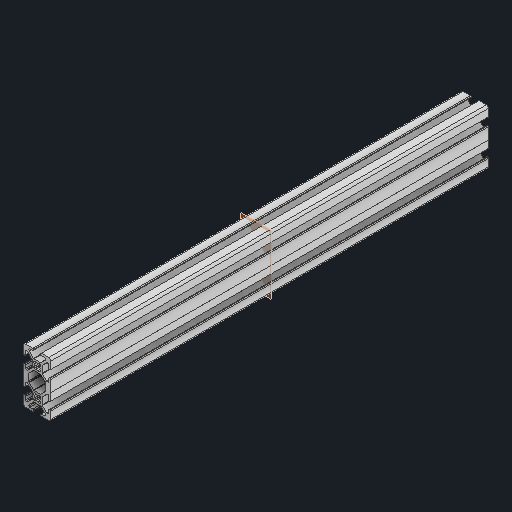
# Autodesk Inventor part: 20-2020-285
Saved by Autodesk Inventor 2026.2 (Build 302298000, 298)
## iProperties
Created: 2024-06-13
Part Number: 20-2020-285
Material: Generic
Document SubType Name: Modeling
Designer: mumin
Density: 1 g/cm^3
Appearance: Default
Author: mumin
Autodesk Inventor part; units mm, degrees
ref_plane "YZ Plane" through (0, 0, 0) normal (1, 0, 0) x (0, 1, 0)
ref_plane "XZ Plane" through (0, 0, 0) normal (0, 1, 0) x (-1, 0, 0)
sketch "Sketch1" plane through (0, 0, 0) normal (0, 0, 1) x (1, 0, 0)
  arc A0 (-10, -8.5) -> (-8.5, -10) centre (-8.5, -8.5) ccw
  line L0 (-8.5, -10) -> (-3.138, -10)
  arc A1 (-3.138, -10) -> (-2.63, -9.492) centre (-3.138, -9.492) ccw
  line L1 (-2.63, -9.492) -> (-2.63, -9.008)
  arc A2 (-2.63, -9.008) -> (-3.138, -8.5) centre (-3.138, -9.008) ccw
  line L2 (-3.138, -8.5) -> (-5.487, -8.5)
  arc A3 (-5.995, -7.992) -> (-5.487, -8.5) centre (-5.487, -7.992) ccw
  line L3 (-5.995, -7.992) -> (-5.995, -7.2662)
  arc A4 (-5.8462, -6.907) -> (-5.995, -7.2662) centre (-5.487, -7.2662) ccw
  line L4 (-5.8462, -6.907) -> (-2.743, -3.8038)
  arc A5 (-2.3838, -3.655) -> (-2.743, -3.8038) centre (-2.3838, -4.163) ccw
  line L5 (-2.3838, -3.655) -> (2.3841, -3.655)
  arc A6 (2.7433, -3.8038) -> (2.3841, -3.655) centre (2.3841, -4.163) ccw
  line L6 (2.7433, -3.8038) -> (5.8462, -6.9067)
  arc A7 (5.995, -7.2659) -> (5.8462, -6.9067) centre (5.487, -7.2659) ccw
  line L7 (5.995, -7.2659) -> (5.995, -7.992)
  arc A8 (5.487, -8.5) -> (5.995, -7.992) centre (5.487, -7.992) ccw
  line L8 (5.487, -8.5) -> (3.138, -8.5)
  arc A9 (3.138, -8.5) -> (2.63, -9.008) centre (3.138, -9.008) ccw
  line L9 (2.63, -9.008) -> (2.63, -9.492)
  arc A10 (2.63, -9.492) -> (3.138, -10) centre (3.138, -9.492) ccw
  line L10 (3.138, -10) -> (8.5, -10)
  arc A11 (8.5, -10) -> (10, -8.5) centre (8.5, -8.5) ccw
  line L11 (10, -8.5) -> (10, -3.138)
  arc A12 (10, -3.138) -> (9.492, -2.63) centre (9.492, -3.138) ccw
  line L12 (9.492, -2.63) -> (9.008, -2.63)
  arc A13 (9.008, -2.63) -> (8.5, -3.138) centre (9.008, -3.138) ccw
  line L13 (8.5, -3.138) -> (8.5, -5.487)
  arc A14 (7.992, -5.995) -> (8.5, -5.487) centre (7.992, -5.487) ccw
  line L14 (7.992, -5.995) -> (7.2662, -5.995)
  arc A15 (6.907, -5.8462) -> (7.2662, -5.995) centre (7.2662, -5.487) ccw
  line L15 (6.907, -5.8462) -> (3.8038, -2.743)
  arc A16 (3.655, -2.3838) -> (3.8038, -2.743) centre (4.163, -2.3838) ccw
  line L16 (3.655, -2.3838) -> (3.655, 2.3841)
  arc A17 (3.8038, 2.7433) -> (3.655, 2.3841) centre (4.163, 2.3841) ccw
  line L17 (3.8038, 2.7433) -> (6.9067, 5.8462)
  arc A18 (7.2659, 5.995) -> (6.9067, 5.8462) centre (7.2659, 5.487) ccw
  line L18 (7.2659, 5.995) -> (7.992, 5.995)
  arc A19 (8.5, 5.487) -> (7.992, 5.995) centre (7.992, 5.487) ccw
  line L19 (8.5, 5.487) -> (8.5, 3.138)
  arc A20 (8.5, 3.138) -> (9.008, 2.63) centre (9.008, 3.138) ccw
  line L20 (9.008, 2.63) -> (9.492, 2.63)
  arc A21 (9.492, 2.63) -> (10.0003, 3.1379) centre (9.4923, 3.138) ccw
  line L21 (10.0003, 3.1379) -> (10.0003, 8.4999)
  line L22 (5.995, 12.0036) -> (5.995, 7.2663)
  arc A22 (5.8462, 6.9071) -> (5.995, 7.2663) centre (5.487, 7.2663) ccw
  line L23 (5.8462, 6.9071) -> (2.7429, 3.8038)
  arc A23 (2.3837, 3.655) -> (2.7429, 3.8038) centre (2.3837, 4.163) ccw
  line L24 (2.3837, 3.655) -> (-2.3841, 3.655)
  arc A24 (-2.7433, 3.8038) -> (-2.3841, 3.655) centre (-2.3841, 4.163) ccw
  line L25 (-2.7433, 3.8038) -> (-5.8462, 6.9067)
  arc A25 (-5.995, 7.2659) -> (-5.8462, 6.9067) centre (-5.487, 7.2659) ccw
  line L26 (-5.995, 7.2659) -> (-5.995, 7.992)
  arc A26 (-5.995, 7.9973) -> (-5.995, 7.992) centre (-5.487, 7.992) ccw
  line L27 (-10, 16.8673) -> (-10, 3.138)
  arc A27 (-10, 3.138) -> (-9.492, 2.63) centre (-9.492, 3.138) ccw
  line L28 (-9.492, 2.63) -> (-9.008, 2.63)
  arc A28 (-9.008, 2.63) -> (-8.5, 3.138) centre (-9.008, 3.138) ccw
  line L29 (-8.5, 3.138) -> (-8.5, 5.487)
  arc A29 (-7.992, 5.995) -> (-8.5, 5.487) centre (-7.992, 5.487) ccw
  line L30 (-7.992, 5.995) -> (-7.2662, 5.995)
  arc A30 (-6.907, 5.8462) -> (-7.2662, 5.995) centre (-7.2662, 5.487) ccw
  line L31 (-6.907, 5.8462) -> (-3.8038, 2.743)
  arc A31 (-3.655, 2.3838) -> (-3.8038, 2.743) centre (-4.163, 2.3838) ccw
  line L32 (-3.655, 2.3838) -> (-3.655, -2.3841)
  arc A32 (-3.8038, -2.7433) -> (-3.655, -2.3841) centre (-4.163, -2.3841) ccw
  line L33 (-3.8038, -2.7433) -> (-6.9067, -5.8462)
  arc A33 (-7.2659, -5.995) -> (-6.9067, -5.8462) centre (-7.2659, -5.487) ccw
  line L34 (-7.2659, -5.995) -> (-7.992, -5.995)
  arc A34 (-8.5, -5.487) -> (-7.992, -5.995) centre (-7.992, -5.487) ccw
  line L35 (-8.5, -5.487) -> (-8.5, -3.138)
  arc A35 (-8.5, -3.138) -> (-9.008, -2.63) centre (-9.008, -3.138) ccw
  line L36 (-9.008, -2.63) -> (-9.492, -2.63)
  arc A36 (-9.492, -2.63) -> (-10, -3.138) centre (-9.492, -3.138) ccw
  line L37 (-10, -3.138) -> (-10, -8.5)
  arc A37 (-1.9358, -0.8037) -> (-2.3045, -2.1245) centre (-1.748, -1.568) ccw
  line L38 (-2.3045, -2.1245) -> (-2.1245, -2.3045)
  arc A38 (-2.1245, -2.3045) -> (-0.8037, -1.9358) centre (-1.568, -1.748) ccw
  arc A39 (-0.8037, -1.9358) -> (0.8037, -1.9358) centre (0, 0) ccw
  arc A40 (0.8037, -1.9358) -> (2.1245, -2.3045) centre (1.568, -1.748) ccw
  line L39 (2.1245, -2.3045) -> (2.3045, -2.1245)
  arc A41 (2.3045, -2.1245) -> (1.9358, -0.8037) centre (1.748, -1.568) ccw
  arc A42 (1.9358, -0.8037) -> (1.9358, 0.8037) centre (0, 0) ccw
  arc A43 (1.9358, 0.8037) -> (2.3045, 2.1245) centre (1.748, 1.568) ccw
  line L40 (2.3045, 2.1245) -> (2.1245, 2.3045)
  arc A44 (2.1245, 2.3045) -> (0.8037, 1.9358) centre (1.568, 1.748) ccw
  arc A45 (0.8037, 1.9358) -> (-0.8037, 1.9358) centre (0, 0) ccw
  arc A46 (-0.8037, 1.9358) -> (-2.1245, 2.3045) centre (-1.568, 1.748) ccw
  line L41 (-2.1245, 2.3045) -> (-2.3045, 2.1245)
  arc A47 (-2.3045, 2.1245) -> (-1.9358, 0.8037) centre (-1.748, 1.568) ccw
  arc A48 (-1.9358, 0.8037) -> (-1.9358, -0.8037) centre (0, 0) ccw
  arc A49 (-8.5, 14.513) -> (-7.992, 14.005) centre (-7.992, 14.513) ccw
  line L42 (-7.2659, 14.005) -> (-7.992, 14.005)
  arc A50 (-7.2659, 14.005) -> (-6.9067, 14.1538) centre (-7.2659, 14.513) ccw
  line L43 (-5.995, 7.9973) -> (-5.995, 12.7338)
  arc A51 (-5.8462, 13.093) -> (-5.995, 12.7338) centre (-5.487, 12.7338) ccw
  line L44 (-3.8038, 17.2567) -> (-6.9067, 14.1538)
  line L45 (-5.8462, 13.093) -> (-2.743, 16.1962)
  arc A52 (-8.5, 16.862) -> (-9.008, 17.37) centre (-9.008, 16.862) ccw
  arc A53 (-9.492, 17.37) -> (-10, 16.862) centre (-9.492, 16.862) ccw
  line L46 (-9.008, 17.37) -> (-9.492, 17.37)
  line L47 (-8.5, 14.513) -> (-8.5, 16.862)
  arc A54 (2.7433, 16.1962) -> (2.3841, 16.345) centre (2.3841, 15.837) ccw
  line L48 (2.7433, 16.1962) -> (5.8462, 13.0933)
  arc A55 (5.995, 12.7341) -> (5.8462, 13.0933) centre (5.487, 12.7341) ccw
  line L49 (5.995, 12.7341) -> (5.995, 12.008)
  line L50 (7.992, 14.005) -> (7.2662, 14.005)
  arc A56 (6.907, 14.1538) -> (7.2662, 14.005) centre (7.2662, 14.513) ccw
  line L51 (6.907, 14.1538) -> (3.8038, 17.257)
  arc A57 (7.992, 14.005) -> (8.5, 14.513) centre (7.992, 14.513) ccw
  line L52 (10, 8.5313) -> (10, 16.862)
  arc A58 (9.008, 17.37) -> (8.5, 16.862) centre (9.008, 16.862) ccw
  line L53 (9.492, 17.37) -> (9.008, 17.37)
  arc A59 (10, 16.862) -> (9.492, 17.37) centre (9.492, 16.862) ccw
  line L54 (8.5, 16.862) -> (8.5, 14.513)
  arc A60 (5.995, 12.0027) -> (5.995, 12.008) centre (5.487, 12.008) ccw
  arc A61 (-2.3838, 16.345) -> (-2.743, 16.1962) centre (-2.3838, 15.837) ccw
  line L55 (-2.3838, 16.345) -> (2.3841, 16.345)
  line L56 (2.1245, 17.6946) -> (2.3045, 17.8746)
  arc A62 (2.3045, 17.8746) -> (1.9358, 19.1953) centre (1.748, 18.4311) ccw
  arc A63 (0.8037, 18.0633) -> (2.1245, 17.6946) centre (1.568, 18.2511) ccw
  arc A64 (-0.8037, 18.0633) -> (0.8037, 18.0633) centre (0, 19.9991) ccw
  line L57 (-2.3045, 17.8746) -> (-2.1245, 17.6946)
  arc A65 (-1.9358, 19.1953) -> (-2.3045, 17.8746) centre (-1.748, 18.4311) ccw
  arc A66 (-2.1245, 17.6946) -> (-0.8037, 18.0633) centre (-1.568, 18.2511) ccw
  arc A67 (2.63, 29.008) -> (3.138, 28.5) centre (3.138, 29.008) ccw
  arc A68 (3.138, 30) -> (2.63, 29.492) centre (3.138, 29.492) ccw
  line L58 (2.63, 29.492) -> (2.63, 29.008)
  arc A69 (3.8038, 22.7433) -> (3.655, 22.3841) centre (4.163, 22.3841) ccw
  arc A70 (2.3837, 23.655) -> (2.7429, 23.8038) centre (2.3837, 24.163) ccw
  line L59 (3.8038, 22.7433) -> (6.9067, 25.8462)
  arc A71 (7.2659, 25.995) -> (6.9067, 25.8462) centre (7.2659, 25.487) ccw
  line L60 (3.138, 28.5) -> (5.487, 28.5)
  arc A72 (5.995, 27.992) -> (5.487, 28.5) centre (5.487, 27.992) ccw
  line L61 (5.995, 27.992) -> (5.995, 27.2662)
  arc A73 (5.8462, 26.907) -> (5.995, 27.2662) centre (5.487, 27.2662) ccw
  line L62 (8.5, 30) -> (3.138, 30)
  arc A74 (10, 28.5) -> (8.5, 30) centre (8.5, 28.5) ccw
  line L63 (7.2659, 25.995) -> (7.992, 25.995)
  arc A75 (8.5, 25.487) -> (7.992, 25.995) centre (7.992, 25.487) ccw
  line L64 (10, 23.138) -> (10, 28.5)
  line L65 (8.5, 25.487) -> (8.5, 23.138)
  line L66 (5.8462, 26.907) -> (2.7429, 23.8038)
  arc A76 (3.655, 17.6162) -> (3.8038, 17.257) centre (4.163, 17.6162) ccw
  line L67 (3.655, 17.6162) -> (3.655, 22.3841)
  line L68 (2.3045, 22.1236) -> (2.1245, 22.3036)
  arc A77 (2.1245, 22.3036) -> (0.8037, 21.9349) centre (1.568, 21.7471) ccw
  arc A78 (1.9358, 20.8028) -> (2.3045, 22.1236) centre (1.748, 21.5671) ccw
  arc A79 (0.8037, 21.9349) -> (-0.8037, 21.9349) centre (0, 19.9991) ccw
  arc A80 (1.9358, 19.1953) -> (1.9358, 20.8028) centre (0, 19.9991) ccw
  line L69 (2.3837, 23.655) -> (-2.3841, 23.655)
  line L70 (-2.7433, 23.8038) -> (-5.8462, 26.9067)
  arc A81 (-5.995, 27.2659) -> (-5.8462, 26.9067) centre (-5.487, 27.2659) ccw
  line L71 (-5.995, 27.2659) -> (-5.995, 27.992)
  arc A82 (-6.9071, 25.8462) -> (-7.2663, 25.995) centre (-7.2663, 25.487) ccw
  arc A83 (-7.992, 25.995) -> (-8.5, 25.487) centre (-7.992, 25.487) ccw
  line L72 (-6.9071, 25.8462) -> (-3.8038, 22.743)
  line L73 (-10, 28.5) -> (-10, 23.138)
  line L74 (-8.5, 23.138) -> (-8.5, 25.487)
  arc A84 (-9.008, 22.63) -> (-8.5, 23.138) centre (-9.008, 23.138) ccw
  line L75 (-9.492, 22.63) -> (-9.008, 22.63)
  arc A85 (-10, 23.138) -> (-9.492, 22.63) centre (-9.492, 23.138) ccw
  line L76 (-7.992, 25.995) -> (-7.2663, 25.995)
  arc A86 (-5.487, 28.5) -> (-5.995, 27.992) centre (-5.487, 27.992) ccw
  arc A87 (-8.5, 30) -> (-10, 28.5) centre (-8.5, 28.5) ccw
  line L77 (-3.138, 30) -> (-8.5, 30)
  line L78 (-5.487, 28.5) -> (-3.138, 28.5)
  arc A88 (-2.7433, 23.8038) -> (-2.3841, 23.655) centre (-2.3841, 24.163) ccw
  arc A89 (-3.655, 22.3838) -> (-3.8038, 22.743) centre (-4.163, 22.3838) ccw
  arc A90 (-3.138, 28.5) -> (-2.63, 29.008) centre (-3.138, 29.008) ccw
  line L79 (-2.63, 29.008) -> (-2.63, 29.492)
  arc A91 (-2.63, 29.492) -> (-3.138, 30) centre (-3.138, 29.492) ccw
  arc A92 (-3.8038, 17.2567) -> (-3.655, 17.6159) centre (-4.163, 17.6159) ccw
  arc A93 (8.5, 23.138) -> (9.008, 22.63) centre (9.008, 23.138) ccw
  line L80 (9.008, 22.63) -> (9.492, 22.63)
  arc A94 (9.492, 22.63) -> (10, 23.138) centre (9.492, 23.138) ccw
  line L81 (-2.1245, 22.3036) -> (-2.3045, 22.1236)
  arc A95 (-2.3045, 22.1236) -> (-1.9358, 20.8028) centre (-1.748, 21.5671) ccw
  arc A96 (-0.8037, 21.9349) -> (-2.1245, 22.3036) centre (-1.568, 21.7471) ccw
  line L82 (-3.655, 22.3838) -> (-3.655, 17.6159)
  arc A97 (-1.9358, 20.8028) -> (-1.9358, 19.1953) centre (0, 19.9991) ccw
  arc A98 (-8.8881, 9.9489) -> (-8.8884, 9.9489) centre (-8.5, 8.5) ccw
  arc A99 (-9.0396, 9.8996) -> (-9.0401, 9.8994) centre (-8.5, 8.5) ccw
  arc A100 (-9.9489, 11.1119) -> (-9.9489, 11.1117) centre (-8.5, 11.5) ccw
  arc A101 (-9.8996, 10.9604) -> (-9.8994, 10.9599) centre (-8.5, 11.5) ccw
  arc A102 (-9.8994, 9.0401) -> (-9.8996, 9.0396) centre (-8.5, 8.5) ccw
  arc A103 (-9.9489, 8.8884) -> (-9.9489, 8.8881) centre (-8.5, 8.5) ccw
  arc A104 (-9.0401, 10.1006) -> (-9.0396, 10.1004) centre (-8.5, 11.5) ccw
  arc A105 (-8.8884, 10.0511) -> (-8.8881, 10.0511) centre (-8.5, 11.5) ccw
  line L83 (-8.4935, 10) -> (-8.5, 10)
  line L84 (-8.5, 10) -> (-8.4935, 10)
  arc A106 (8.8884, 9.9489) -> (8.8881, 9.9489) centre (8.5004, 8.4999) ccw
  arc A107 (9.0401, 9.8994) -> (9.0396, 9.8996) centre (8.5004, 8.4999) ccw
  arc A108 (10, 11.4908) -> (10, 11.5) centre (8.5, 11.5) ccw
  arc A109 (10.0003, 8.4999) -> (10, 8.5327) centre (8.5004, 8.4999) ccw
  line L85 (-3.655, 19.9998) -> (3.655, 20.0002)
  point P0 (0, 0)
  point P1 (3.655, 10)
  point P2 (3.655, 8.5)
  point P3 (-10, 8.5)
  constraints: 224 point on circle, 172 end point, 110 centre point, 28 point on line, 2 midpoint
extrude "Extrusion1" add sketch "Sketch1" along normal mid plane 320 contours L37 A36 L36 A35 L35 A34 L34 A33 L33 A32 L32 A31 L31 A30 L30 A29 L29 A28 L28 A27 L27 A98 A100 A53 L46 A52 L47 A49 L42 A50 L44 A92 L82 L85 A97 A65 L57 A66 A64 A63 L56 A62 A80 L67 A76 L51 A56 L50 A57 L54 A58 L53 A59 L52 A106 L21 A21 L20 A20 L19 A19 L18 A18 L17 A17 L16 A16 L15 A15 L14 A14 L13 A13 L12 A12 L11 A11 L10 A10 L9 A9 L8 A8 L7 A7 L6 A6 L5 A5 L4 A4 L3 A3 L2 A2 L1 A1 L0 A0 | L27 A100 A98 | A98 | A100 A98 | L82 A89 L72 A82 L76 A83 L74 A84 L75 A85 L73 A87 L77 A91 L79 A90 L78 A86 L71 A81 L70 A88 L69 A70 L66 A73 L61 A72 L60 A67 L58 A68 L62 A74 L64 A94 L80 A93 L65 A75 L63 A71 L59 A69 L67 L85 A80 A78 L68 A77 A79 A96 L81 A95 A97 | A106
body "Solid1"
